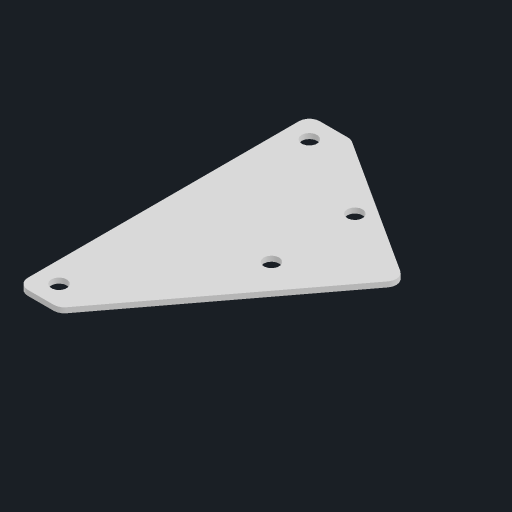
# Autodesk Inventor part: andrewSled
Saved by Autodesk Inventor 2024.2 (Build 282272000, 272)
## iProperties
Created: 2024-01-22
Part Number: andrewSled
Material: Generic
Document SubType Name: Sheet Metal
Designer: reima
Density: 1 g/cm^3
Sheet Metal Rule: Default
Appearance: Default
Author: reima
Autodesk Inventor part; units mm, degrees
ref_plane "YZ Plane" through (0, 0, 0) normal (1, 0, 0) x (0, 1, 0)
ref_plane "XZ Plane" through (0, 0, 0) normal (0, 1, 0) x (-1, 0, 0)
ref_plane "XY Plane" through (0, 0, 0) normal (0, 0, 1) x (1, 0, 0)
sketch "Sketch1" plane through (0, 0, 0) normal (0, 1, 0) x (-1, 0, 0)
  circle A0 centre (0, 0) radius 2.3368
  circle A1 centre (0, 76.2) radius 2.3368
  circle A2 centre (-26.5684, 12.7) radius 2.3368
  circle A3 centre (-26.5684, 38.1) radius 2.3368
  line L0 (3.175, 82.55) -> (-4.7692, 82.55)
  line L1 (6.35, 82.55) -> (14.2942, 82.55) construction
  line L2 (6.35, 79.375) -> (6.35, -3.175)
  circle A4 centre (-26.5684, -12.7) radius 41.275 construction
  line L3 (-7.3027, 81.2886) -> (-47.1919, 28.4776)
  arc A5 (-4.7692, 82.55) -> (-7.3027, 81.2886) centre (-4.7692, 79.375) ccw
  arc A6 (6.35, 79.375) -> (3.175, 82.55) centre (3.175, 79.375) ccw
  arc A7 (3.175, -6.35) -> (6.35, -3.175) centre (3.175, -3.175) ccw
  line L4 (-5.4147, -6.35) -> (3.175, -6.35)
  line L5 (-7.1359, -5.843) -> (-48.6254, 20.9227)
  line L6 (-49.4377, 25.5043) -> (-47.1919, 28.4776)
  arc A8 (-49.4377, 25.5043) -> (-48.6254, 20.9227) centre (-46.9042, 23.5907) ccw
  arc A9 (-7.1359, -5.843) -> (-5.4147, -6.35) centre (-5.4147, -3.175) ccw
  point P0 (-6.35, 82.55)
  point P1 (-6.35, -6.35)
  point P2 (6.35, -6.35)
  point P3 (-67.352, -6.35)
  dimension "d17" = 82.55
  dimension "d0" = 4.6736
  dimension "d2" = 76.2
  dimension "d3" = 4.6736
  dimension "d4" = 4.6736
  dimension "d5" = 4.6736
  dimension "d6" = 12.7
  dimension "d7" = 26.5684
  dimension "d8" = 25.4
  dimension "d9" = 0
  dimension "d10" = 12.7
  dimension "d11" = 180
  dimension "d12" = 6.35
  dimension "d13" = 6.35
  dimension "d14" = 12.7
  dimension "d15" = 6.35
  dimension "d16" = 6.35
  dimension "d18" = 25.4
  dimension "d19" = 0
  dimension "d20" = 3.175
  dimension "d22" = 9.525
  dimension "d23" = 3.175
  measures "d0" diameter of A0
  measures "d2" distance of point (0, 0) A1.centre
  measures "d3" diameter of A1
  measures "d4" diameter of A2
  measures "d5" diameter of A3
  measures "d6" vertical distance of point (0, 0) A2.centre
  measures "d7" horizontal distance of point (0, 0) A2.centre
  measures "d8" distance of A2.centre A3.centre
  measures "d9" horizontal distance of A2.centre A3.centre
  measures "d10" distance of L1.start point (-6.35, 82.55)
  measures "d11" angle of L0 L1
  measures "d12" distance from line of L0 A1.centre
  measures "d13" horizontal distance of A1.centre L1.start
  measures "d14" distance of point (-6.35, -6.35) point (6.35, -6.35)
  measures "d15" horizontal distance of point (0, 0) point (6.35, -6.35)
  measures "d16" horizontal distance of point (0, 0) point (6.35, -6.35)
  measures "d18" distance of point (-26.568, -12.7) A2.centre
  measures "d19" horizontal distance of point (-26.568, -12.7) A2.centre
  measures "d20" radius of A5
  measures "d22" distance of point (-6.35, -6.35) L4.end
  measures "d23" radius of A8
extrude "Plate1" add sketch "Sketch1" along normal blind 1.5875
equation "\"d21\" = Thickness"
equation "\"BendRadius\" = Thickness"
equation "\"BendReliefWidth\" = Thickness"
equation "\"BendReliefDepth\" = 0.5 * Thickness"
equation "\"CornerReliefSize\" = 4 * Thickness"
equation "\"MinimumRemnant\" = 2 * Thickness"
equation "\"TransitionRadius\" = BendRadius"
equation "\"JacobiRadiusSize\" = BendRadius"
equation "\"GapSize\" = Thickness"
equation "\"Thickness\" = 1.5875"
body "Solid1"
